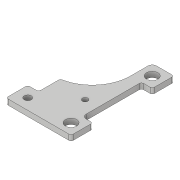
# Autodesk Inventor part: autodesk
Saved by Autodesk Inventor 2019 (Build 230136000, 136)
## iProperties
Created: 2020-02-08
Part Number: autodesk
Material: Generic
Document SubType Name: Modeling
Designer: risha
Density: 1 g/cm^3
Appearance: Default
Author: risha
Autodesk Inventor part; units mm, degrees
ref_plane "YZ Plane" through (0, 0, 0) normal (1, 0, 0) x (0, 1, 0)
ref_plane "XZ Plane" through (0, 0, 0) normal (0, 1, 0) x (-1, 0, 0)
ref_plane "XY Plane" through (0, 0, 0) normal (0, 0, 1) x (1, 0, 0)
sketch "Sketch1" plane through (0, 0, 0) normal (0, 1, 0) x (-1, 0, 0)
  line L0 (3.9336, 17.4729) -> (3.9336, -2.5271)
  line L1 (3.9336, -2.5271) -> (13.9336, -2.5271)
  line L2 (13.9336, -2.5271) -> (13.9336, -57.5271)
  line L3 (13.9336, -57.5271) -> (3.9336, -57.5271)
  line L4 (3.9336, -57.5271) -> (3.9336, -77.5271)
  line L5 (3.9336, -77.5271) -> (23.9336, -77.5271)
  line L6 (23.9336, -77.5271) -> (23.9336, -57.5271)
  line L7 (3.9336, 17.4729) -> (63.9336, 17.4729)
  line L8 (63.9336, 17.4729) -> (63.9336, -2.5271)
  line L9 (63.9336, -2.5271) -> (53.9336, -2.5271)
  line L10 (53.9336, -2.5271) -> (53.9336, -22.5271)
  arc A0 (53.9336, -22.5271) -> (23.9336, -57.5271) centre (59.3503, -57.5271) ccw
  point P0 (0, 0)
  dimension "d0" = 20
  dimension "d1" = 10
  dimension "d2" = 55
  dimension "d3" = 10
  dimension "d4" = 20
  dimension "d5" = 20
  dimension "d6" = 20
  dimension "d7" = 60
  dimension "d8" = 20
  dimension "d9" = 10
  dimension "d10" = 20
  constraints: 22 end point, 6 perpendicular, 3 vertical, 2 horizontal, 2 point on circle, 1 centre point, 1 tangent
  measures "d0" distance of L0.start L0.end
  measures "d1" distance of L0.end L1.end
  measures "d2" distance of L1.end L2.end
  measures "d3" distance of L2.end L3.end
  measures "d4" distance of L3.end L4.end
  measures "d5" distance of L4.end L5.end
  measures "d6" distance of L5.end L6.end
  measures "d7" distance of L0.start L7.end
  measures "d8" distance of L7.end L8.end
  measures "d9" distance of L8.end L9.end
  measures "d10" distance of L9.end L10.end
extrude "Extrusion1" add sketch "Sketch1" along normal blind 5
sketch "Sketch2" plane through (0, 5, 0) normal (0, 1, 0) x (1, 0, 0)
  circle A0 centre (-13.9336, -7.4729) radius 5.25
  circle A1 centre (-13.9336, 67.5271) radius 5.25
  circle A2 centre (-53.9336, -7.4729) radius 3.25
  point P0 (0, 0)
  point P1 (-3.9336, -17.4729)
  point P2 (-3.9336, 77.5271)
  dimension "d15" = 10.5
  dimension "d18" = 10.5
  dimension "d21" = 6.5
  constraints: 3 centre point
  measures "d15" diameter of A0
  measures "d18" diameter of A1
  measures "d21" diameter of A2
extrude "Extrusion2" cut sketch "Sketch2" along normal through all both and the other way through all
sketch "Sketch3" plane through (0, 5, 0) normal (0, 1, 0) x (1, 0, 0)
  line L0 (-63.9336, -17.4729) -> (-3.9336, -17.4729) projected
  line L1 (-13.9336, 2.5271) -> (-13.9336, 57.5271) projected
  circle A0 centre (-25.9336, 17.5271) radius 2.5
  point P0 (0, 0)
  dimension "d27" = 5
  constraints: 1 centre point
  measures "d27" diameter of A0
extrude "Extrusion3" cut sketch "Sketch3" against normal through all
fillet "Fillet1" radius 4 2 edges at (-13.9336, 2.5, -2.5271) (-23.9336, 2.5, -77.5271)
fillet "Fillet2" radius 2 7 edges at (-3.9336, 2.5, 17.4729) (-63.9336, 2.5, 17.4729) (-3.9336, 2.5, -2.5271) (-3.9336, 2.5, -57.5271) (-3.9336, 2.5, -77.5271) (-63.9336, 2.5, -2.5271) (-53.9336, 2.5, -22.5271)
fillet "Fillet3" radius 2 2 edges at (-13.9336, 2.5, -57.5271) (-53.9336, 2.5, -2.5271)
body "Solid1"
